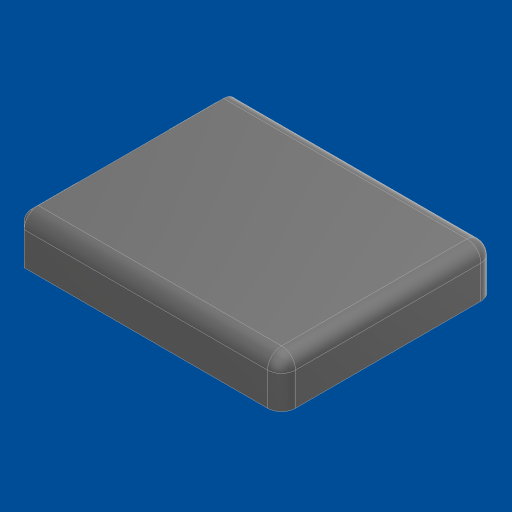
# Autodesk Inventor part: aus-200_top
Saved by Autodesk Inventor 2023.2 (Build 272271000, 271)
## iProperties
Created: 2023-01-27
Part Number: aus-200_top
Material: PC/ABS Plastic
Document SubType Name: Modeling
Designer: agmlego
Mass: 3.83671 g
Surface Area: 154.602 cm^2
Volume: 10.7389 cm^3
Density: 0.357273 g/cm^3
Appearance: Smooth - Black
Author: agmlego
Autodesk Inventor part; units mm, degrees
ref_plane "YZ Plane" through (0, 0, 0) normal (1, 0, 0) x (0, 1, 0)
ref_plane "XZ Plane" through (0, 0, 0) normal (0, 1, 0) x (-1, 0, 0)
ref_plane "XY Plane" through (0, 0, 0) normal (0, 0, 1) x (1, 0, 0)
sketch "Sketch1" plane through (0, 0, 0) normal (1, 0, 0) x (0, 1, 0)
  line L0 (6.72, 30.5) -> (-6.72, 30.5)
  line L1 (-6.72, 30.5) -> (-6.72, -30.5)
  line L2 (-6.72, -30.5) -> (6.72, -30.5)
  line L3 (6.72, -30.5) -> (6.72, 30.5)
  line L4 (6.72, 0) -> (-6.72, 0) construction
  point P0 (0, 0)
  point P1 (0, 0)
  dimension "d0" = 61
  dimension "d1" = 13.44
  constraints: 10 end point, 3 midpoint, 2 parallel, 1 coincident, 1 horizontal, 1 perpendicular
  measures "d0" distance between parallel lines of L2 L0
  measures "d1" distance between parallel lines of L1 L3
extrude "Extrusion1" add sketch "Sketch1" along normal blind 75.6
sketch "Sketch2" plane through (0, -6.72, -30.5) normal (0, -1, 0) x (1, 0, 0)
  line L0 (1.54, 1.5) -> (74, 1.5)
  line L1 (74, 1.5) -> (74, 59.5)
  line L2 (74, 59.5) -> (1.54, 59.5)
  line L3 (1.54, 59.5) -> (1.54, 1.5)
  line L4 (0, 30.5) -> (1.54, 30.5) construction
  line L5 (0, 61) -> (0, 0) construction
  line L6 (75.6, 61) -> (75.6, 0) construction
  line L7 (0, 61) -> (75.6, 61) construction
  dimension "d4" = 1.54
  dimension "d5" = 1.6
  dimension "d6" = 1.5
  constraints: 10 end point, 2 parallel, 2 perpendicular, 1 horizontal, 1 midpoint
  measures "d4" distance between parallel lines of L5 L3
  measures "d5" distance between parallel lines of L6 L1
  measures "d6" distance between parallel lines of L7 L2
extrude "Extrusion2" cut sketch "Sketch2" against normal blind 12.02
fillet "Fillet1" radius 4 5 edges at (37.8, 6.72, -30.5) (75.6, 6.72, 0) (75.6, 0, -30.5) (37.8, 6.72, 30.5) (75.6, 0, 30.5)
fillet "Fillet2" radius 2.4 5 edges at (74, -0.71, -29) (37.77, 5.3, -29) (74, 5.3, 0) (74, -0.71, 29) (37.77, 5.3, 29)
sketch "Sketch3" plane through (0, 0, 0) normal (-1, 0, 0) x (0, 0, 1)
  line L0 (-30.5, -6.72) -> (-30.5, 2.72) projected
  arc A0 (-26.5, 6.72) -> (-30.5, 2.72) centre (-26.5, 2.72) ccw projected
  line L1 (-26.5, 6.72) -> (26.5, 6.72) projected
  arc A1 (30.5, 2.72) -> (26.5, 6.72) centre (26.5, 2.72) ccw projected
  line L2 (30.5, 2.72) -> (30.5, -6.72) projected
  line L3 (28.55, -6.72) -> (28.55, 2.72)
  arc A2 (28.55, 2.72) -> (26.5, 4.77) centre (26.5, 2.72) ccw
  line L4 (26.5, 4.77) -> (-26.5, 4.77)
  arc A3 (-26.5, 4.77) -> (-28.55, 2.72) centre (-26.5, 2.72) ccw
  line L5 (-28.55, 2.72) -> (-28.55, -6.72)
  line L6 (-26.5, -6.72) -> (-30.5, -6.72) construction
  line L7 (-28.55, -6.72) -> (-30.5, -6.72)
  line L8 (28.55, -6.72) -> (30.5, -6.72)
  line L9 (-29, -6.72) -> (29, -6.72) construction
  point P0 (0, 0)
  dimension "d11" = 1.95
  constraints: 10 end point, 4 point on circle, 2 centre point, 2 collinear, 4 other
  measures "d11" distance between parallel lines of L1 L4
extrude "Extrusion3" cut sketch "Sketch3" against normal blind 2
sketch "Sketch4" plane through (1.54, -6.72, 28.55) normal (1, 0, 0) x (0, 0, -1)
  line L0 (1.95, 12.02) -> (55.15, 12.02) projected
  arc A0 (57.55, 9.62) -> (55.15, 12.02) centre (55.15, 9.62) ccw projected
  line L1 (57.55, 9.62) -> (57.55, 0) projected
  arc A1 (1.95, 12.02) -> (-0.45, 9.62) centre (1.95, 9.62) ccw projected
  line L2 (-0.45, 0) -> (-0.45, 9.62) projected
  line L3 (56.55, 0) -> (56.55, 9.62)
  arc A2 (56.55, 9.62) -> (55.15, 11.02) centre (55.15, 9.62) ccw
  line L4 (55.15, 11.02) -> (1.95, 11.02)
  arc A3 (1.95, 11.02) -> (0.55, 9.62) centre (1.95, 9.62) ccw
  line L5 (0.55, 9.62) -> (0.55, 0)
  line L6 (56.55, 0) -> (57.55, 0)
  line L7 (-0.45, 0) -> (0.55, 0)
  line L8 (57.1, 0) -> (0, 0) construction
  point P0 (28.55, 6.72)
  dimension "d14" = 1
  constraints: 10 end point, 4 point on circle, 2 centre point, 1 collinear, 1 perpendicular, 4 other
  measures "d14" distance between parallel lines of L1 L3
extrude "Extrusion4" add sketch "Sketch4" along normal blind 1
sketch "Sketch5" plane through (0, 0, 0) normal (-1, 0, 0) x (0, 0, 1)
  arc A0 (-26.5, 6.72) -> (-30.5, 2.72) centre (-26.5, 2.72) ccw projected
  line L0 (-26.5, 6.72) -> (26.5, 6.72) projected
  line L1 (-30.5, -6.72) -> (-30.5, 2.72) projected
  line L2 (-29, -6.72) -> (-30.5, -6.72) projected
  line L3 (-28.55, -6.72) -> (-29, -6.72) projected
  line L4 (-28.55, 2.72) -> (-28.55, -6.72) projected
  arc A1 (-26.5, 4.77) -> (-28.55, 2.72) centre (-26.5, 2.72) ccw projected
  line L5 (26.5, 4.77) -> (-26.5, 4.77) projected
  arc A2 (30.5, 2.72) -> (26.5, 6.72) centre (26.5, 2.72) ccw projected
  arc A3 (28.55, 2.72) -> (26.5, 4.77) centre (26.5, 2.72) ccw projected
  line L6 (28.55, -6.72) -> (28.55, 2.72) projected
  line L7 (30.5, 2.72) -> (30.5, -6.72) projected
  line L8 (30.5, -6.72) -> (29, -6.72) projected
  line L9 (29, -6.72) -> (28.55, -6.72) projected
  point P0 (0, 0)
extrude "Extrusion5" cut sketch "Sketch5" against normal up to surface (2 mm away)
sketch "Sketch6" plane through (0, 0, 0) normal (-1, 0, 0) x (0, 0, 1)
  line L0 (26.5, 4.77) -> (-26.5, 4.77) construction
  line L1 (-13, 4.77) -> (13, 4.77)
  line L2 (13, 4.77) -> (13, 3.82)
  line L3 (13, 3.82) -> (-13, 3.82)
  line L4 (-13, 3.82) -> (-13, 4.77)
  line L5 (-26.5, 6.72) -> (26.5, 6.72) construction
  point P0 (0, 0)
  point P1 (0, 4.77)
  dimension "d19" = 26
  dimension "d21" = 2.9
  constraints: 8 end point, 2 midpoint, 2 parallel, 1 horizontal, 1 perpendicular, 1 point on line
  measures "d19" distance of L2.end L3.end
  measures "d21" distance between parallel lines of L3 L5
extrude "Extrusion6" cut sketch "Sketch6" against normal up to surface (2 mm away)
sketch "Sketch7" plane through (0, 0, 0) normal (-1, 0, 0) x (0, 0, 1)
  line L0 (-5.925, 1.32) -> (5.925, 1.32)
  line L1 (5.925, 1.32) -> (5.925, 4.52)
  line L2 (5.925, 4.52) -> (-5.925, 4.52)
  line L3 (-5.925, 4.52) -> (-5.925, 1.32)
  line L4 (-26.5, 6.72) -> (26.5, 6.72) construction
  line L5 (0, 6.72) -> (0, 4.52) construction
  point P0 (0, 0)
  dimension "d24" = 2.2
  dimension "d25" = 3.2
  dimension "d26" = 11.85
  constraints: 10 end point, 2 midpoint, 2 parallel, 2 perpendicular, 1 horizontal
  measures "d24" distance between parallel lines of L4 L2
  measures "d25" distance of L2.end L0.start
  measures "d26" distance of L0.start L0.end
extrude "Extrusion7" cut sketch "Sketch7" against normal up to surface (2.54 mm away)
sketch "Sketch8" plane through (0, 0, 0) normal (-1, 0, 0) x (0, 0, 1)
  line L0 (-19.935, -6.72) -> (19.935, -6.72)
  line L1 (19.935, -6.72) -> (19.935, -9.05)
  line L2 (19.935, -9.05) -> (-19.935, -9.05)
  line L3 (-19.935, -9.05) -> (-19.935, -6.72)
  line L4 (28.55, -6.72) -> (-28.55, -6.72) construction
  point P0 (0, 0)
  point P1 (0, -6.72)
  dimension "d29" = 39.87
  dimension "d30" = 2.33
  constraints: 8 end point, 2 midpoint, 2 parallel, 1 horizontal, 1 perpendicular
  measures "d29" distance of L1.end L2.end
  measures "d30" distance of L2.end L0.start
extrude "Extrusion8" add sketch "Sketch8" against normal up to surface (1.54 mm away)
sketch "Sketch9" plane through (0, 0, 0) normal (-1, 0, 0) x (0, 0, 1)
  line L0 (-21.185, 0.16) -> (-19.935, 0.16)
  line L1 (-19.935, 0.16) -> (-19.935, -6.72)
  line L2 (-19.935, -6.72) -> (-21.185, -6.72)
  line L3 (-21.185, -6.72) -> (-21.185, 0.16)
  line L4 (19.935, 0.16) -> (21.185, 0.16)
  line L5 (21.185, 0.16) -> (21.185, -6.72)
  line L6 (21.185, -6.72) -> (19.935, -6.72)
  line L7 (19.935, -6.72) -> (19.935, 0.16)
  line L8 (-19.935, -3.28) -> (19.935, -3.28) construction
  line L9 (0, 0) -> (0, -3.28) construction
  line L10 (-19.935, -6.72) -> (-19.935, -9.05) construction
  line L11 (-19.935, -6.72) -> (-28.55, -6.72) construction
  dimension "d33" = 1.25
  dimension "d34" = 6.88
  constraints: 20 end point, 4 parallel, 4 perpendicular, 3 midpoint, 2 collinear, 2 equal length, 2 horizontal
  measures "d33" distance of L0.start L0.end
  measures "d34" distance of L2.end L0.start
extrude "Extrusion9" cut sketch "Sketch9" against normal blind 0.85
body "Solid1"
